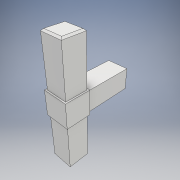
# Autodesk Inventor part: Profile-Connector#04
Saved by Autodesk Inventor 2018 (Build 220112000, 112)
## iProperties
Created: 2025-02-16
Part Number: Profile-Connector#04
Material: PVC potrubí
Document SubType Name: Modeling
Designer: Jozko Mrkvicka
Density: 1.4 g/cm^3
Appearance: Hladká – bílá
Author: Jozko Mrkvicka
Autodesk Inventor part; units mm, degrees
ref_plane "YZ Plane" through (0, 0, 0) normal (1, 0, 0) x (0, 1, 0)
ref_plane "XZ Plane" through (0, 0, 0) normal (0, 1, 0) x (-1, 0, 0)
ref_plane "XY Plane" through (0, 0, 0) normal (0, 0, 1) x (1, 0, 0)
sketch "Náčrt8" plane through (0, 0, 0) normal (0, 1, 0) x (-1, 0, 0)
  line L0 (-15, 15) -> (15, 15)
  line L1 (15, 15) -> (15, -15)
  line L2 (15, -15) -> (-15, -15)
  line L3 (-15, -15) -> (-15, 15)
  line L4 (-15, 15) -> (15, -15) construction
  line L5 (15, 15) -> (-15, -15) construction
  point P0 (0, 0)
  dimension "d67" = 30
  dimension "d68" = 30
  constraints: 12 end point, 2 midpoint, 2 parallel, 1 horizontal, 1 perpendicular
  measures "d67" distance of L1.end L2.end
  measures "d68" distance of L0.end L1.end
extrude "Vysunutí8" add sketch "Náčrt8" along normal blind 30
sketch "Náčrt9" plane through (0, 30, 0) normal (0, 1, 0) x (1, 0, 0)
  line L0 (13, -13) -> (-13, -13)
  line L1 (-13, -13) -> (-13, 13)
  line L2 (-13, 13) -> (13, 13)
  line L3 (13, 13) -> (13, -13)
  line L4 (13, -13) -> (-13, 13) construction
  line L5 (-13, -13) -> (13, 13) construction
  point P0 (0, 0)
  dimension "d71" = 26
  dimension "d72" = 26
  constraints: 12 end point, 2 midpoint, 2 parallel, 1 horizontal, 1 perpendicular
  measures "d71" distance of L1.end L2.end
  measures "d72" distance of L0.end L1.end
extrude "Vysunutí9" add sketch "Náčrt9" along normal blind 60
sketch "Náčrt10" plane through (-15, 0, -15) normal (-1, 0, 0) x (0, 0, 1)
  line L0 (30, 0) -> (0, 0) projected
  line L1 (30, 0) -> (30, 30) projected
  line L2 (0, 30) -> (30, 30) projected
  line L3 (0, 0) -> (0, 30) projected
  line L4 (28, 2) -> (2, 2)
  line L5 (2, 2) -> (2, 28)
  line L6 (2, 28) -> (28, 28)
  line L7 (28, 28) -> (28, 2)
  line L8 (28, 2) -> (2, 28) construction
  line L9 (2, 2) -> (28, 28) construction
  point P0 (15, 0)
  point P1 (7.5, 15)
  point P2 (15, 15)
  dimension "d79" = 26
  dimension "d80" = 26
  dimension "d120" = 15
  dimension "d121" = 15
  constraints: 12 end point, 2 midpoint, 2 parallel, 1 horizontal, 1 perpendicular
  measures "d79" distance of L5.end L6.end
  measures "d80" distance of L4.end L5.end
  measures "d120" distance from line of L3 point (15, 15)
  measures "d121" distance from line of L2 point (15, 15)
sketch "Náčrt11" plane through (15, 0, -15) normal (0, 0, -1) x (-1, 0, 0)
  line L0 (30, 0) -> (0, 0) projected
  line L1 (30, 0) -> (30, 30) projected
  line L2 (0, 30) -> (30, 30) projected
  line L3 (0, 0) -> (0, 30) projected
  line L4 (28, 2) -> (2, 2)
  line L5 (2, 2) -> (2, 28)
  line L6 (2, 28) -> (28, 28)
  line L7 (28, 28) -> (28, 2)
  line L8 (28, 2) -> (2, 28) construction
  line L9 (2, 2) -> (28, 28) construction
  point P0 (15, 0)
  point P1 (15, 15)
  dimension "d87" = 26
  dimension "d88" = 26
  dimension "d122" = 15
  dimension "d123" = 15
  constraints: 12 end point, 2 midpoint, 2 parallel, 1 horizontal, 1 perpendicular
  measures "d87" distance of L5.end L6.end
  measures "d88" distance of L4.end L5.end
  measures "d122" distance from line of L2 point (15, 15)
  measures "d123" distance from line of point (15, 15) L3
sketch "Náčrt12" plane through (15, 0, 15) normal (1, 0, 0) x (0, 0, -1)
  line L0 (2, 2) -> (28, 2) projected
  line L1 (28, 28) -> (2, 28) projected
  line L2 (28, 2) -> (28, 28) projected
  line L3 (2, 28) -> (2, 2) projected
  point P0 (15, 0)
sketch "Náčrt13" plane through (0, 0, 0) normal (0, -1, 0) x (1, 0, 0)
  line L0 (13, -13) -> (13, 13) projected
  line L1 (-13, -13) -> (13, -13) projected
  line L2 (-15, 15) -> (15, 15) projected
  line L3 (13, 13) -> (-13, 13) projected
  line L4 (-13, 13) -> (-13, -13) projected
sketch "Náčrt14" plane through (-15, 0, 15) normal (0, 0, 1) x (1, 0, 0)
  line L0 (28, 28) -> (2, 28) projected
  line L1 (2, 28) -> (2, 2) projected
  line L2 (2, 2) -> (28, 2) projected
  line L3 (28, 2) -> (28, 28) projected
  point P0 (15, 0)
extrude "Vysunutí10" add sketch "Náčrt11" along normal blind 60 contours L4 L5 L6 L7
extrude "Vysunutí11" add sketch "Náčrt14" along normal blind 60
extrude "Vysunutí12" [suppressed]
extrude "Vysunutí13" [suppressed]
extrude "Vysunutí14" [suppressed]
chamfer "Zkosení13" [suppressed]
chamfer "Zkosení14" distance 2 angle 45 4 edges at (13, 15, -75) (-13, 15, -75) (0, 28, -75) (0, 2, -75)
chamfer "Zkosení15" [suppressed]
chamfer "Zkosení16" distance 2 angle 45 4 edges at (-13, 15, 75) (13, 15, 75) (0, 28, 75) (0, 2, 75)
chamfer "Zkosení17" distance 2 angle 45 4 edges at (-13, 90, 0) (0, 90, -13) (13, 90, 0) (0, 90, 13)
chamfer "Zkosení18" [suppressed]
equation "\"d67\" = width"
equation "\"d68\" = width"
equation "\"d69\" = width"
equation "\"d71\" = width - 2 * thickness"
equation "\"d72\" = width - 2 * thickness"
equation "\"d75\" = 2 * width"
equation "\"d79\" = width - 2 * thickness"
equation "\"d80\" = width - 2 * thickness"
equation "\"d120\" = 0.5 * width"
equation "\"d121\" = 0.5 * width"
equation "\"d87\" = width - 2 * thickness"
equation "\"d88\" = width - 2 * thickness"
equation "\"d122\" = 0.5 * width"
equation "\"d123\" = 0.5 * width"
equation "\"d89\" = 2 * width"
equation "\"d91\" = 2 * width"
equation "\"d93\" = 2 * width"
equation "\"d95\" = 2 * width"
equation "\"d97\" = 2 * width"
equation "\"d99\" = thickness"
equation "\"d102\" = thickness"
equation "\"d105\" = thickness"
equation "\"d108\" = thickness"
equation "\"d111\" = thickness"
equation "\"d114\" = thickness"
equation "\"width\" = 30"
equation "\"thickness\" = 2"
